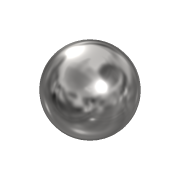
# Autodesk Inventor part: Ш.02.Шарик 4
Saved by Autodesk Inventor 2021.3 (Build 253353010, 353A)
## iProperties
Created: 2021-07-07
Part Number: Ш.02.Шарик 4
Material: Stainless Steel
Document SubType Name: Modeling
Designer: Михальчик
Density: 8 g/cm^3
Appearance: Semi-Polished
Author: Михальчик
Autodesk Inventor part; units mm, degrees
ref_plane "YZ Plane" through (0, 0, 0) normal (1, 0, 0) x (0, 1, 0)
ref_plane "XZ Plane" through (0, 0, 0) normal (0, 1, 0) x (-1, 0, 0)
ref_plane "XY Plane" through (0, 0, 0) normal (0, 0, 1) x (1, 0, 0)
sketch "Sketch1" plane through (0, 0, 0) normal (1, 0, 0) x (0, 1, 0)
  circle A0 centre (0, 0) radius 2
  line L0 (-2, 0) -> (2, 0)
  dimension "d0" = 4
  dimension "d0" = 4
  constraints: 2 end point, 2 point on circle, 1 centre point, 1 coincident
  measures "d0" diameter of A0
revolve "Revolution1" add sketch "Sketch1" angle 360 about axis through (0, -2, 0) along (0, 1, 0) picked at (-0.5903, -0.3098) contours A0 L0
body "Solid1"
